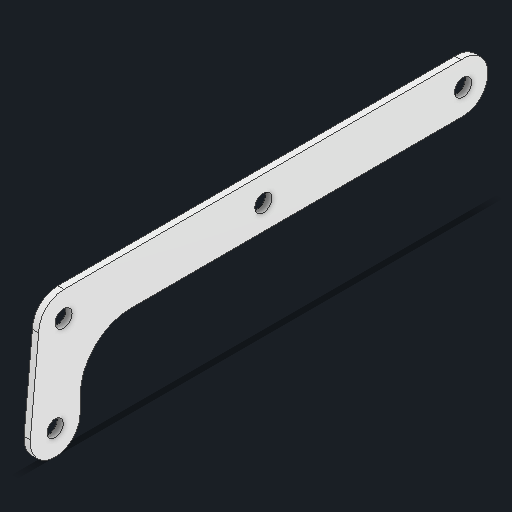
# Autodesk Inventor part: Passive Gusset
Saved by Autodesk Inventor 2025.1 (Build 291241000, 241)
## iProperties
Created: 2024-10-24
Part Number: Passive Gusset
Material: Acetal Resin, White
Document SubType Name: Sheet Metal
Designer: avere
Density: 1.425 g/cm^3
Appearance: Smooth - White
Mass: 1.90026 g
Surface Area: 27.8658 cm^2
Volume: 1.90026 cm^3
Flat Pattern Width: 3.58438 cm
Flat Pattern Length: 11.6455 cm
Flat Pattern Area: 41.7417 cm^2
Sheet Metal Rule: Default_mm
Sheet Metal Width: 1.411 in
Sheet Metal Length: 4.585 in
Sheet Metal Area: 6.470 in^2
d0: 0.500 in
d1: 0.500 in
d2: 0.500 in
d3: 0.165 in
d7: 0.172 in
d8: 0.172 in
d9: 0.500 in
Author: avere
Autodesk Inventor part; units mm, degrees
ref_plane "YZ Plane" through (0, 0, 0) normal (1, 0, 0) x (0, 1, 0)
ref_plane "XZ Plane" through (0, 0, 0) normal (0, 1, 0) x (-1, 0, 0)
ref_plane "XY Plane" through (0, 0, 0) normal (0, 0, 1) x (1, 0, 0)
sketch "main" plane through (0, 0, 0) normal (0, 0, 1) x (1, 0, 0)
  circle A0 centre (33.3097, -13.5548) radius 2.1844
  arc A1 (33.2126, -19.9041) -> (39.6597, -13.5466) centre (33.3097, -13.5548) ccw
  arc A2 (41.7862, 8.9717) -> (29.1145, 9.6144) centre (35.4643, 9.5687) ccw
  line L0 (39.6597, -13.5466) -> (41.7862, 8.9717)
  line L1 (-68.2903, -7.2251) -> (16.3844, -7.2251)
  line L2 (29.0841, 5.3837) -> (29.1145, 9.6144)
  arc A3 (16.3844, -7.2251) -> (29.0841, 5.3837) centre (16.3844, 5.4749) ccw
  circle A4 centre (35.4643, 9.5687) radius 2.0955
  line L3 (33.4068, -19.9041) -> (-67.7743, -19.9041)
  circle A5 centre (-68.2903, -13.5751) radius 2.1844
  circle A6 centre (-17.4821, -13.5224) radius 2.1844
  arc A7 (-68.2903, -7.2251) -> (-67.7743, -19.9041) centre (-68.2903, -13.5751) ccw
  point P0 (20.4908, -8.19)
  dimension "d0" = 12.7
  dimension "d1" = 12.7
  dimension "d2" = 12.7
  dimension "d3" = 4.191
  dimension "d7" = 4.3688
  dimension "d8" = 4.3688
  dimension "d9" = 12.7
  measures "d0" diameter of A1
  measures "d1" diameter of A2
  measures "d2" radius of A3
  measures "d3" diameter of A4
  measures "d7" diameter of A5
  measures "d8" diameter of A0
  measures "d9" diameter of A7
sketch "Sketch1" plane through (0, 0, 0) normal (1, 0, 0) x (0, 1, 0)
  circle A0 centre (-0.0052, 63.4918) radius 2.1844
  arc A1 (6.3442, 63.3994) -> (-0.0181, 69.8418) centre (-0.0052, 63.4918) ccw
  arc A2 (-22.538, 71.9516) -> (-23.1712, 59.2794) centre (-23.1303, 65.6293) ccw
  line L0 (-0.0181, 69.8418) -> (-22.538, 71.9516)
  line L1 (-6.2598, -38.1129) -> (-6.3224, 46.5618)
  line L2 (-18.9405, 59.2522) -> (-23.1712, 59.2794)
  arc A3 (-6.3224, 46.5618) -> (-18.9405, 59.2522) centre (-19.0224, 46.5524) ccw
  circle A4 centre (-23.1303, 65.6293) radius 2.0955
  line L3 (6.344, 63.5936) -> (6.4188, -37.5875)
  circle A5 centre (0.0902, -38.1082) radius 2.1844
  circle A6 centre (0, 12.7) radius 2.1844
  arc A7 (-6.2598, -38.1129) -> (6.4188, -37.5875) centre (0.0902, -38.1082) ccw
  point P0 (0, 0)
extrude "Extrusion1" add sketch "Sketch1" along normal blind 1.5875
equation "\"BendRadius\" = Thickness"
equation "\"BendReliefWidth\" = Thickness"
equation "\"BendReliefDepth\" = 0.5 * Thickness"
equation "\"CornerReliefSize\" = 4 * Thickness"
equation "\"MinimumRemnant\" = 2 * Thickness"
equation "\"TransitionRadius\" = BendRadius"
equation "\"JacobiRadiusSize\" = BendRadius"
equation "\"GapSize\" = Thickness"
equation "\"Thickness\" = 1.5875"
body "Solid1"
